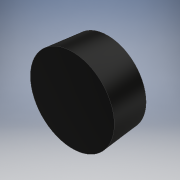
# Autodesk Inventor part: Base
Saved by Autodesk Inventor 2017 (Build 210142000, 142)
## iProperties
Created: 2018-10-14
Part Number: Base
Material: Generic
Document SubType Name: Modeling
Designer: Cameron
Density: 1 g/cm^3
Appearance: Glossy - Black
Author: Cameron
Autodesk Inventor part; units mm, degrees
ref_plane "YZ Plane" through (0, 0, 0) normal (1, 0, 0) x (0, 1, 0)
ref_plane "XY Plane" through (0, 0, 0) normal (0, 0, 1) x (1, 0, 0)
sketch "Sketch1" plane through (0, 0, 0) normal (0, 1, 0) x (-1, 0, 0)
  circle A0 centre (0, 0) radius 47.5
  dimension "d0" = 95
  constraints: 1 centre point, 1 coincident
  measures "d0" diameter of A0
ref_plane "Work Plane1" through (0, 40, 0) normal (0, 1, 0) x (-1, 0, 0)
sketch "Sketch2" plane through (0, 40, 0) normal (0, 1, 0) x (-1, 0, 0)
  circle A0 centre (0, 0) radius 43.5
  dimension "d2" = 87
  constraints: 1 centre point, 1 coincident
  measures "d2" diameter of A0
loft "Loft1" add profiles "Sketch1", "Sketch2"
body "Solid1"
